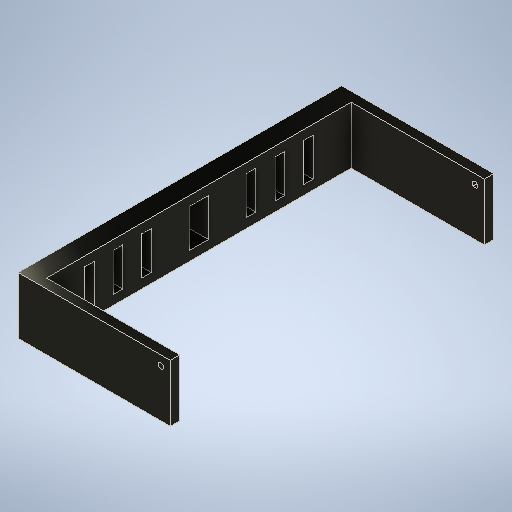
# Autodesk Inventor part: BONNET
Saved by Autodesk Inventor 2025.3 (Build 293356030, 356C)
## iProperties
Created: 2026-06-30
Part Number: BONNET
Material: ABS Plastic
Document SubType Name: Modeling
Designer: user
Density: 1.06 g/cm^3
Appearance: Gunmetal
Author: user
Autodesk Inventor part; units mm, degrees
ref_plane "YZ Plane" through (0, 0, 0) normal (1, 0, 0) x (0, 1, 0)
ref_plane "XZ Plane" through (0, 0, 0) normal (0, 1, 0) x (-1, 0, 0)
ref_plane "XY Plane" through (0, 0, 0) normal (0, 0, 1) x (1, 0, 0)
sketch "Sketch1" plane through (0, 0, 0) normal (1, 0, 0) x (0, 1, 0)
  line L0 (0, 0) -> (30, 0)
  line L1 (30, 0) -> (30, -160)
  line L2 (30, -160) -> (0, -160)
  line L3 (0, -160) -> (0, 0)
  line L4 (25, -20) -> (5, -20)
  line L5 (0, -20) -> (0, -25)
  line L6 (5, -25) -> (25, -25)
  line L7 (30, -25) -> (30, -20)
  line L8 (25, -35) -> (5, -35)
  line L9 (0, -35) -> (0, -40)
  line L10 (5, -40) -> (25, -40)
  line L11 (30, -40) -> (30, -35)
  line L12 (25, -50) -> (5, -50)
  line L13 (0, -50) -> (0, -55)
  line L14 (5, -55) -> (25, -55)
  line L15 (30, -55) -> (30, -50)
  line L16 (25, -75) -> (5, -75)
  line L17 (0, -75) -> (0, -85)
  line L18 (5, -85) -> (25, -85)
  line L19 (30, -85) -> (30, -75)
  line L20 (25, -105) -> (5, -105)
  line L21 (0, -105) -> (0, -110)
  line L22 (5, -110) -> (25, -110)
  line L23 (30, -110) -> (30, -105)
  line L24 (25, -120) -> (5, -120)
  line L25 (0, -120) -> (0, -125)
  line L26 (5, -125) -> (25, -125)
  line L27 (30, -125) -> (30, -120)
  line L28 (25, -135) -> (5, -135)
  line L29 (0, -135) -> (0, -140)
  line L30 (5, -140) -> (25, -140)
  line L31 (30, -140) -> (30, -135)
  line L32 (30, 0) -> (25, 0)
  line L33 (25, 0) -> (25, -160)
  line L34 (25, -160) -> (30, -160)
  line L35 (30, -160) -> (30, 0)
  line L36 (0, 0) -> (5, 0)
  line L37 (5, 0) -> (5, -160)
  line L38 (5, -160) -> (0, -160)
  line L39 (0, -160) -> (0, 0)
  line L40 (30, 0) -> (0, 0)
  line L41 (0, 0) -> (0, 5)
  line L42 (0, 5) -> (30, 5)
  line L43 (30, 5) -> (30, 0)
  line L44 (30, -160) -> (0, -160)
  line L45 (0, -160) -> (0, -165)
  line L46 (0, -165) -> (30, -165)
  line L47 (30, -165) -> (30, -160)
  dimension "d0" = 30
  dimension "d1" = 160
  dimension "d2" = 5
  dimension "d3" = 20
  dimension "d4" = 5
  dimension "d5" = 5
  dimension "d6" = 10
  dimension "d7" = 5
  dimension "d8" = 5
  dimension "d9" = 5
  dimension "d10" = 20
  dimension "d12" = 10
  dimension "d14" = 20
  dimension "d15" = 10
  dimension "d16" = 10
  dimension "d17" = 10
  dimension "d18" = 5
  dimension "d19" = 5
  dimension "d20" = 5
  dimension "d21" = 5
  constraints: 88 end point, 21 parallel, 15 horizontal, 9 perpendicular, 3 point on line, 2 vertical, 54 other
  measures "d0" distance of L2.start L2.end
  measures "d1" distance of L0.end L2.start
  measures "d2" distance of L5.end L5.start
  measures "d3" distance between parallel lines of L4 L0
  measures "d4" distance of L9.end L9.start
  measures "d5" distance of L13.end L13.start
  measures "d6" distance of L17.end L17.start
  measures "d7" distance of L21.end L21.start
  measures "d8" distance of L25.end L25.start
  measures "d9" distance of L29.end L29.start
  measures "d10" distance between parallel lines of L2 L30
  measures "d12" distance between parallel lines of L12 L10
  measures "d14" distance between parallel lines of L20 L18
  measures "d15" distance between parallel lines of L24 L22
  measures "d16" distance between parallel lines of L28 L26
  measures "d17" distance between parallel lines of L6 L8
  measures "d18" distance of L34.end L34.start
  measures "d19" distance of L38.start L38.end
  measures "d20" distance of L40.end L41.end
  measures "d21" distance of L45.end L44.end
extrude "Extrusion1" add sketch "Sketch1" along normal blind 10 contours L0 L37 L2 L3 | L0 L33 L4 L37 | L0 L1 L2 L33 | L6 L33 L8 L37 | L10 L33 L12 L37 | L14 L33 L16 L37 | L18 L33 L20 L37 | L22 L33 L24 L37 | L26 L33 L28 L37 | L30 L33 L2 L37
extrude "Extrusion2" add sketch "Sketch1" along normal blind 80 contours L41 L42 L43 L0 | L2 L47 L46 L45
sketch "Sketch2" plane through (0, 0, 5) normal (0, 0, 1) x (1, 0, 0)
  line L0 (80, 30) -> (80, 0) projected
  line L1 (0, 0) -> (80, 0) projected
  point P0 (75, 25)
  dimension "d33" = 5
  dimension "d34" = 25
  measures "d33" distance from line of L0 point (75, 25)
  measures "d34" distance from line of L1 point (75, 25)
hole "Hole1" at (75, 25, 5) direction (0, 0, -1) diameter 3 end through all
body "Solid1"
